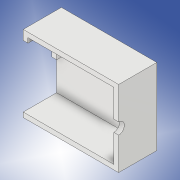
# Autodesk Inventor part: FA001
Saved by Autodesk Inventor 2017 SP1 (Build 210196100, 196)
## iProperties
Created: 2017-06-16
Part Number: FA001
Material: ABS Plastic
Document SubType Name: Modeling
Designer: Zach
Density: 1.06 g/cm^3
Appearance: CR White
Author: Zach
Autodesk Inventor part; units mm, degrees
ref_plane "YZ Plane" through (0, 0, 0) normal (1, 0, 0) x (0, 1, 0)
ref_plane "XZ Plane" through (0, 0, 0) normal (0, 1, 0) x (-1, 0, 0)
ref_plane "XY Plane" through (0, 0, 0) normal (0, 0, 1) x (1, 0, 0)
sketch "Sketch1" plane through (0, 0, 0) normal (0, 0, 1) x (1, 0, 0)
  line L0 (0, 0) -> (100, 0)
  line L1 (100, 0) -> (100, 80)
  line L2 (100, 80) -> (0, 80)
  line L3 (0, 80) -> (0, 0)
  dimension "d0" = 100
  dimension "d1" = 80
  constraints: 8 end point, 2 parallel, 1 horizontal, 1 perpendicular
  measures "d0" distance of L2.end L1.end
  measures "d1" distance of L1.end L0.end
extrude "Extrusion1" add sketch "Sketch1" along normal blind 40
sketch "Sketch2" plane through (0, 0, 40) normal (0, 0, 1) x (1, 0, 0)
  line L0 (100, 80) -> (0, 80) projected
  line L1 (100, 0) -> (100, 80) projected
  line L2 (0, 0) -> (100, 0) projected
  line L3 (0, 75) -> (95, 75)
  line L4 (95, 75) -> (95, 5)
  line L5 (95, 5) -> (0, 5)
  line L6 (0, 75) -> (0, 5)
  line L7 (0, 80) -> (0, 0) projected
  dimension "d4" = 5
  constraints: 8 end point, 1 collinear, 2 other
  measures "d4" distance between parallel lines of L0 L3
extrude "Extrusion2" cut sketch "Sketch2" against normal blind 35 contours L3 L4 L5 L6
sketch "Sketch3" plane through (0, 0, 0) normal (-1, 0, 0) x (0, 0, 1)
  line L0 (0, 80) -> (40, 80) projected
  line L1 (0, 0) -> (40, 0) projected
  line L2 (0, 80) -> (10, 80)
  line L3 (10, 80) -> (10, 40)
  line L4 (10, 40) -> (0, 40)
  line L5 (0, 40) -> (0, 80)
  line L6 (40, 75) -> (40, 5) projected
  line L7 (0, 80) -> (40, 80)
  line L8 (40, 80) -> (40, 70)
  line L9 (40, 70) -> (0, 70)
  line L10 (0, 70) -> (0, 80)
  dimension "d7" = 10
  dimension "d8" = 10
  dimension "d11" = 40
  constraints: 16 end point, 4 parallel, 2 horizontal, 2 perpendicular, 1 point on line
  measures "d7" distance of L3.end L4.end
  measures "d8" distance of L7.end L8.end
  measures "d11" vertical distance of L1.end L3.end
extrude "Extrusion3" add sketch "Sketch3" against normal blind 5
sketch "Sketch4" plane through (100, 0, 0) normal (1, 0, 0) x (0, 0, -1)
  line L0 (-40, 75) -> (-40, 5) projected
  circle A0 centre (-40, 40) radius 6
  point P0 (0, 0)
  dimension "d12" = 12
  constraints: 1 centre point, 1 midpoint
  measures "d12" diameter of A0
extrude "Extrusion4" cut sketch "Sketch4" against normal through all
body "Solid1"
